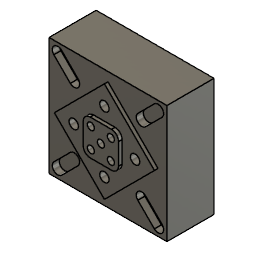
CNC MILING (Autodesk Fusion 360 design; units mm, degrees)
part number: 2026-05-19-10-16-22-673
Autodesk Fusion 360 part; units mm, degrees
sketch "Sketch1" plane through (0, 0, 0) normal (0, 0, 1) x (1, 0, 0)
  line L0 (-25, 25) -> (25, 25)
  line L1 (25, 25) -> (25, -25)
  line L2 (25, -25) -> (-25, -25)
  line L3 (-25, -25) -> (-25, 25)
  line L4 (-25, 25) -> (25, -25) construction
  line L5 (25, 25) -> (-25, -25) construction
  dimension "d1" = 50
  dimension "d2" = 50
  constraint horizontal L0
  constraint perpendicular L0 L1
  constraint parallel L0 L2
  constraint parallel L1 L3
  constraint coincident L4 origin
  constraint coincident L5 origin
  measures "d1" distance of L0.start L0.end
  measures "d2" distance of L0.end L1.end
extrude "Extrude1" add sketch "Sketch1" along normal blind 20
sketch "Sketch2" plane through (0, 0, 20) normal (0, 0, 1) x (1, 0, 0)
  line L0 (-25, -25) -> (25, -25)
  line L1 (25, -25) -> (25, 25)
  line L2 (25, 25) -> (-25, 25)
  line L3 (-25, 25) -> (-25, -25)
  line L4 (21.2132, 0) -> (0, -21.2132)
  line L5 (0, -21.2132) -> (-21.2132, 0)
  line L6 (-21.2132, 0) -> (0, 21.2132)
  line L7 (0, 21.2132) -> (21.2132, 0)
  line L8 (0, -25) -> (0, 25) construction
  line L9 (0, -21.2132) -> (0, 21.2132) construction
  line L10 (21.2132, 0) -> (-21.2132, 0) construction
  line L11 (25, 0) -> (-25, 0) construction
  dimension "d5" = 30
  dimension "d6" = 30
  constraint perpendicular L4 L5
  constraint perpendicular L5 L6
  constraint perpendicular L4 L7
  constraint midpoint L0 L8.start
  constraint midpoint L2 L8.end
  constraint vertical L9
  constraint midpoint L1 L11.start
  constraint midpoint L3 L11.end
  constraint collinear L8 L9
  constraint collinear L10 L11
  measures "d5" distance of L5.end L6.end
  measures "d6" distance of L4.end L5.end
extrude "Extrude2" add sketch "Sketch2" along normal blind 1.5 contours L4 L5 L6 L7
sketch "Sketch3" plane through (0, 0, 21.5) normal (0, 0, 1) x (1, 0, 0)
  line L0 (0, 21.2132) -> (-21.2132, 0)
  line L1 (-21.2132, 0) -> (0, -21.2132)
  line L2 (0, -21.2132) -> (21.2132, 0)
  line L3 (21.2132, 0) -> (0, 21.2132)
  circle A0 centre (0, 0) radius 13 construction
  circle A1 centre (0, -13) radius 2.5
  circle A2 centre (-13, 0) radius 2.5
  circle A3 centre (0, 13) radius 2.5
  circle A4 centre (13, 0) radius 2.5
  dimension "d9" = 26
  dimension "d10" = 5
  constraint coincident A0.centre origin
  constraint coincident A0 A1.centre
  constraint coincident A0 A2.centre
  constraint coincident A0 A3.centre
  constraint coincident A0 A4.centre
  constraint equal A2 A3
  constraint equal A3 A4
  constraint equal A1 A4
  measures "d9" diameter of A0
  measures "d10" diameter of A2
hole "Hole1" at (-13, 0, 21.5) at (0, -13, 21.5) at (0, 13, 21.5) at (13, 0, 21.5) direction (0, 0, -1) diameter 4 depth 3 tip angle 180
sketch "Sketch4" plane through (0, 0, 21.5) normal (0, 0, 1) x (1, 0, 0)
  circle A0 centre (0, 13) radius 2
  circle A1 centre (-13, 0) radius 2
  circle A2 centre (0, -13) radius 2
  circle A3 centre (13, 0) radius 2
  line L0 (0, 21.2132) -> (-21.2132, 0)
  line L1 (-21.2132, 0) -> (0, -21.2132)
  line L2 (0, -21.2132) -> (21.2132, 0)
  line L3 (21.2132, 0) -> (0, 21.2132)
  line L4 (4.5, -7.5) -> (-4.5, -7.5)
  line L5 (-7.5, -4.5) -> (-7.5, 4.5)
  line L6 (-4.5, 7.5) -> (4.5, 7.5)
  line L7 (7.5, 4.5) -> (7.5, -4.5)
  line L8 (7.5, -7.5) -> (-7.5, 7.5) construction
  line L9 (-7.5, -7.5) -> (7.5, 7.5) construction
  arc A4 (4.5, -7.5) -> (7.5, -4.5) centre (4.5, -4.5) ccw
  arc A5 (-7.5, -4.5) -> (-4.5, -7.5) centre (-4.5, -4.5) ccw
  arc A6 (7.5, 4.5) -> (4.5, 7.5) centre (4.5, 4.5) ccw
  arc A7 (-4.5, 7.5) -> (-7.5, 4.5) centre (-4.5, 4.5) ccw
  dimension "d14" = 15
  dimension "d15" = 15
  dimension "d16" = 3
  dimension "d17" = 3
  dimension "d18" = 3
  dimension "d19" = 3
  constraint horizontal L4
  constraint perpendicular L4 L5
  constraint parallel L4 L6
  constraint parallel L5 L7
  constraint coincident L8 origin
  constraint coincident L9 origin
  constraint coincident L8.start L7
  constraint coincident L8.start L4
  constraint tangent L7 A4
  constraint tangent L4 A4
  constraint coincident L9.start L4
  constraint coincident L9.start L5
  constraint tangent L4 A5
  constraint tangent L5 A5
  constraint coincident L9.end L6
  constraint coincident L9.end L7
  constraint tangent L6 A6
  constraint tangent L7 A6
  constraint coincident L8.end L5
  constraint coincident L8.end L6
  constraint tangent L5 A7
  constraint tangent L6 A7
  measures "d14" distance of L8.start L9.start
  measures "d15" distance of L9.start L8.end
  measures "d16" radius of A4
  measures "d17" radius of A5
  measures "d18" radius of A6
  measures "d19" radius of A7
extrude "Extrude3" add sketch "Sketch4" along normal blind 1.5 contours L4 L5 L6 L7 A4 A5 A6 A7
sketch "Sketch5" plane through (0, 0, 23) normal (0, 0, 1) x (1, 0, 0)
  arc A0 (7.5, 4.5) -> (4.5, 7.5) centre (4.5, 4.5) ccw
  line L0 (4.5, 7.5) -> (-4.5, 7.5)
  arc A1 (-4.5, 7.5) -> (-7.5, 4.5) centre (-4.5, 4.5) ccw
  line L1 (-7.5, 4.5) -> (-7.5, -4.5)
  arc A2 (-7.5, -4.5) -> (-4.5, -7.5) centre (-4.5, -4.5) ccw
  line L2 (-4.5, -7.5) -> (4.5, -7.5)
  arc A3 (4.5, -7.5) -> (7.5, -4.5) centre (4.5, -4.5) ccw
  line L3 (7.5, -4.5) -> (7.5, 4.5)
  circle A4 centre (0, 0) radius 6 construction
  line L4 (6.6213, -6.6213) -> (-6.6213, 6.6213) construction
  line L5 (-6.6213, -6.6213) -> (6.6213, 6.6213) construction
  circle A5 centre (0, 0) radius 1.5
  circle A6 centre (-4.2426, -4.2426) radius 1.5
  circle A7 centre (4.2426, -4.2426) radius 1.5
  circle A8 centre (4.2426, 4.2426) radius 1.5
  circle A9 centre (-4.2426, 4.2426) radius 1.5
  dimension "d22" = 12
  dimension "d23" = 3
  constraint coincident A4.centre A5.centre
  constraint midpoint A3 L4.start
  constraint midpoint A1 L4.end
  constraint midpoint A2 L5.start
  constraint midpoint A0 L5.end
  constraint coincident L5 A6.centre
  constraint coincident A4 A6.centre
  constraint coincident L4 A7.centre
  constraint coincident A4 A7.centre
  constraint coincident L5 A8.centre
  constraint coincident A4 A8.centre
  constraint coincident A4 A9.centre
  constraint coincident L4 A9.centre
  constraint equal A6 A9
  constraint equal A8 A9
  constraint equal A7 A8
  constraint equal A5 A7
  measures "d22" diameter of A4
  measures "d23" diameter of A5
hole "Hole2" at (-4.2426, -4.2426, 23) at (4.2426, -4.2426, 23) at (-4.2426, 4.2426, 23) at (4.2426, 4.2426, 23) at (0, 0, 23) direction (0, 0, -1) diameter 3 depth 5 tip angle 180
sketch "Sketch6" plane through (0, 0, 20) normal (0, 0, 1) x (1, 0, 0)
  line L0 (0, 21.2132) -> (21.2132, 0)
  line L1 (21.2132, 0) -> (0, -21.2132)
  line L2 (0, -21.2132) -> (-21.2132, 0)
  line L3 (-21.2132, 0) -> (0, 21.2132)
  line L4 (-25, -25) -> (25, -25)
  line L5 (25, -25) -> (25, 25)
  line L6 (25, 25) -> (-25, 25)
  line L7 (-25, 25) -> (-25, -25)
  line L8 (-25, -25) -> (-10.6066, -10.6066) construction
  line L9 (-19.6648, -22.9418) -> (-12.6648, -15.9418)
  arc A0 (-12.6648, -15.9418) -> (-15.9418, -12.6648) centre (-14.3033, -14.3033) ccw
  line L10 (-15.9418, -12.6648) -> (-22.9418, -19.6648)
  arc A1 (-22.9418, -19.6648) -> (-19.6648, -22.9418) centre (-21.3033, -21.3033) ccw
  line L11 (-21.3033, -21.3033) -> (-14.3033, -14.3033) construction
  line L12 (12.6648, -15.9418) -> (19.6648, -22.9418)
  arc A2 (19.6648, -22.9418) -> (22.9418, -19.6648) centre (21.3033, -21.3033) ccw
  line L13 (22.9418, -19.6648) -> (15.9418, -12.6648)
  arc A3 (15.9418, -12.6648) -> (12.6648, -15.9418) centre (14.3033, -14.3033) ccw
  line L14 (15.9418, 12.6648) -> (22.9418, 19.6648)
  arc A4 (22.9418, 19.6648) -> (19.6648, 22.9418) centre (21.3033, 21.3033) ccw
  line L15 (19.6648, 22.9418) -> (12.6648, 15.9418)
  arc A5 (12.6648, 15.9418) -> (15.9418, 12.6648) centre (14.3033, 14.3033) ccw
  line L16 (-12.6648, 15.9418) -> (-19.6648, 22.9418)
  arc A6 (-19.6648, 22.9418) -> (-22.9418, 19.6648) centre (-21.3033, 21.3033) ccw
  line L17 (-22.9418, 19.6648) -> (-15.9418, 12.6648)
  arc A7 (-15.9418, 12.6648) -> (-12.6648, 15.9418) centre (-14.3033, 14.3033) ccw
  dimension "d28" = 360
  constraint coincident L4.start L7.end
  constraint midpoint L2 L8.end
  constraint tangent L9 A0
  constraint tangent A0 L10
  constraint parallel L9 L10
  constraint tangent L10 A1
  constraint tangent L9 A1
  constraint coincident L8 A0.centre
  constraint parallel L8 L11
  constraint midpoint L8 L11
extrude "Extrude4" cut sketch "Sketch6" against normal blind 3 contours L9 A0 L10 A1 | L12 A2 L13 A3 | L14 A4 L15 A5 | L16 A6 L17 A7
